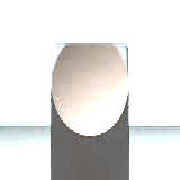
# Autodesk Inventor part: ISO 3601-1 - C 0300 G
Saved by Autodesk Inventor 2021.3 (Build 253353000, 353)
## iProperties
Created: 2020-01-21
Part Number: ISO 3601-1 - C 0300 G
Material: Rubber
Description: Fluid power systems - O-ring
Document SubType Name: Modeling
Standard: ISO 3601-1
Designer: Rémi Heredero
Standard Revision: Third edition 2002-08-01
Standards Organization: ISO
Language: en-US
Size Designation: C 0300 G
Categories: <MemberInstance><Categories><Category DisplayName="Shaft Parts" InternalName="7f7aeb1f-a693-4053-b835-cee3144e0d98" Mnemonic="SHFT"><Category DisplayName="Sealing" InternalName="7cc80d44-b28a-4eb5-95d8-e54d452fb95e" Mnemonic="GSKT"><Category DisplayName="O-Rings" InternalName="33c545bb-13c8-4826-80bf-0503e1d122a8" Mnemonic="ORGSKT"><CategoryParameter DisplayName="O-Ring Inside Diameter" InternalName="2396c6fe-eaf5-4a08-901f-879cfa8d6861" Mnemonic="oindia"/><CategoryParameter DisplayName="O-Ring Cross Section Diameter" InternalName="55cd1771-6829-4a36-adef-b3bef9abff47" Mnemonic="osecdia"/><CategoryParameter DisplayName="Shaft Diameter" InternalName="800cb856-dfd5-475b-a5f5-7930e1c24170" Mnemonic="shaftdia"/><CategoryParameter DisplayName="Thickness" InternalName="d722c673-2dd1-4ecb-b1b2-67404f2aea42" Mnemonic="thick"/><Category DisplayName="Radial Internal" InternalName="94bce4a4-c701-4512-9012-7d41da09bb5a" Mnemonic="ORGSKTRI"><CategoryParameter DisplayName="Groove Width" InternalName="20e3f4bb-a411-4064-be96-21e607b7e471" Mnemonic="NB"/><CategoryParameter DisplayName="Outside Radius" InternalName="58031890-5a64-4422-90a4-8f170607bbac" Mnemonic="R2"/><CategoryParameter DisplayName="Groove Diameter" InternalName="9b90a319-4acb-4bb6-b120-7b7d5fa3e797" Mnemonic="NDOR"/><CategoryParameter DisplayName="Inside Radius" InternalName="cafdab84-b5be-4c6a-8c01-58bfed4b804b" Mnemonic="R1"/></Category></Category></Category></Category><Category DisplayName="DataType" InternalName="23b78d0f-2648-40c6-8793-ca6db495c9e8" Mnemonic="DATATYPE"><CategoryParameter DisplayName="DisplayName" InternalName="05415f3d-3907-474b-a020-eb9d644f4cf3" Mnemonic="DISPLAYNAME"/><CategoryParameter DisplayName="Standard" InternalName="0c0a119c-1e12-4c84-803f-101930972f5e" Mnemonic="STANDARD"/><CategoryParameter DisplayName="Description" InternalName="13903e3d-64b1-4950-80da-f627842ea37f" Mnemonic="DESCRIPTION"/><CategoryParameter DisplayName="Designation" InternalName="2675968c-4ce5-49e0-a4f5-552d29089031" Mnemonic="DESIGNATION"/><CategoryParameter DisplayName="Default Row" InternalName="2af9ec52-faaa-4026-b378-f9fa4afca842" Mnemonic="DEFAULTROW"/><CategoryParameter DisplayName="Folder Name" InternalName="3f06958e-8713-4116-9be7-ed6184ecc97b" Mnemonic="FOLDERNAME"/><CategoryParameter DisplayName="Revision Guid" InternalName="45a75005-10b1-4dfc-8d6d-dfe629f0b93c" Mnemonic="REVISIONGUID"/><CategoryParameter DisplayName="FileName" InternalName="8b46a4cc-9585-4fed-90c3-899f57e09a73" Mnemonic="FILENAME"/><CategoryParameter DisplayName="StdsOrg" InternalName="8f5914e1-4693-403f-8ab5-d37768198c9d" Mnemonic="STDSORG"/><CategoryParameter DisplayName="Family Version" InternalName="914462f6-6e19-4b14-ba84-155b9680b1d0" Mnemonic="FAMILYREVISION"/><CategoryParameter DisplayName="Standard Revision" InternalName="91d5a463-65c2-4fde-b823-3b7fea5e8e17" Mnemonic="STANDARDREVISION"/><CategoryParameter DisplayName="Member Revision" InternalName="a65d44b9-392f-4f4f-857b-e4b3d54996fe" Mnemonic="MEMBERREVISION"/><CategoryParameter DisplayName="ClipFormat" InternalName="bc51e27b-3422-4e78-93ef-cec197ddf230" Mnemonic="CLIPFORMAT"/><CategoryParameter DisplayName="Manufacturer" InternalName="cd6c7a72-a28a-4e50-99a9-2c7f4e13e5ad" Mnemonic="MANUFACTURER"/><CategoryParameter DisplayName="InternalName" InternalName="cf1d0246-76d9-4b4a-8305-fa0409afb5c1" Mnemonic="INTERNALNAME"/><CategoryParameter DisplayName="IsMetric" InternalName="e2385c5b-1ea4-4823-96a8-8de651266ec3" Mnemonic="ISMETRIC"/><Category DisplayName="Part" InternalName="c0e0b642-3bcb-4cc8-9e80-f96d35c4afa4" Mnemonic="PART"><CategoryParameter DisplayName="Part Number" InternalName="016b6077-bfbe-49bd-92c9-d8d59c39c941" Mnemonic="PARTNUMBER"/><CategoryParameter DisplayName="Stock Number" InternalName="4dba7c1c-e26c-444e-836c-b08b433409a8" Mnemonic="STOCKNUMBER"/><CategoryParameter DisplayName="Material Key" InternalName="5c9a8adb-dd2b-4535-b97f-0a94a95fe41f" Mnemonic="MATERIALKEY"/><CategoryParameter DisplayName="Material" InternalName="818a152a-d3c3-49ca-80ee-df7d91421b8e" Mnemonic="MATERIAL"/></Category></Category><Category DisplayName="LegacyMap" InternalName="cd87c42b-3e48-431e-b5c0-1cbeb14dfe77" Mnemonic="LEGACYMAP"><CategoryParameter DisplayName="unique DA member ID" InternalName="0918ad47-427f-4fed-ae26-24c81c58f590" Mnemonic="DACOOKIE"/><CategoryParameter DisplayName="Merge11 ID" InternalName="0ee8fb18-e2ed-4f39-96f6-1f4b5f50aa71" Mnemonic="MERGE11"/><CategoryParameter DisplayName="unique CC member ID" InternalName="5193edd4-b2b0-4ab4-9d54-de900eee34e0" Mnemonic="CCCOOKIE"/><CategoryParameter DisplayName="Split ID" InternalName="72b5c83c-be7f-45c4-ae51-9160ea6deb26" Mnemonic="SPLIT"/><CategoryParameter DisplayName="MemberID" InternalName="8e5e0294-fc51-4c8f-b3d7-003dc5ed94f6" Mnemonic="MEMBERID"/><CategoryParameter DisplayName="CatalogName" InternalName="d99d1e27-aa94-4de2-af4c-c348882a6f4f" Mnemonic="CATALOGNAME"/><CategoryParameter DisplayName="FamilyNumber" InternalName="e705e1f4-09cb-413e-91f9-551b4188271e" Mnemonic="FAMILYNUMBER"/></Category></Categories><FamilyTemplate Id="si0119"><FamilyTemplateParameters><FamilyTemplateParameter ObjectType="kUserParameterObject" ValueType="xs:double" Id="1" ObjectReferenceKey="R1"/><FamilyTemplateParameter ObjectType="kUserParameterObject" ValueType="xs:double" Id="2" ObjectReferenceKey="R2"/><FamilyTemplateParameter ObjectType="kUserParameterObject" ValueType="xs:double" Id="3" ObjectReferenceKey="QDM"/><FamilyTemplateParameter ObjectType="kUserParameterObject" ValueType="xs:double" Id="4" ObjectReferenceKey="SD1"/><FamilyTemplateParameter ObjectType="kUserParameterObject" ValueType="xs:double" Id="5" ObjectReferenceKey="NDOR"/><FamilyTemplateParameter ObjectType="kUserParameterObject" ValueType="xs:double" Id="6" ObjectReferenceKey="NB1"/><FamilyTemplateParameter ObjectType="kUserParameterObject" ValueType="xs:double" Id="7" ObjectReferenceKey="BD"/><FamilyTemplateParameter ObjectType="kUserParameterObject" ValueType="xs:double" Id="8" ObjectReferenceKey="NND"/><FamilyTemplateParameter ObjectType="kUserParameterObject" ValueType="xs:double" Id="120" ObjectReferenceKey="NTOR"/><FamilyTemplateParameter ObjectType="kPropertyObject" ValueType="xs:string" Id="100" ObjectReferenceKey="{32853F0F-3444-11d1-9E93-0060B03C1CA6}" SubObjectId="52"/><FamilyTemplateParameter ObjectType="kPropertyObject" ValueType="xs:string" Id="105" ObjectReferenceKey="{32853F0F-3444-11d1-9E93-0060B03C1CA6}" SubObjectId="5"/><FamilyTemplateParameter ObjectType="kPartComponentDefinitionObject" ValueType="xs:string" Id="110" SubObjectId="Material"/></FamilyTemplateParameters></FamilyTemplate><CategoryParameterMap><ParamToTemplateMap><ParamToTemplate CategoryParameter="//CategoryParameter[@InternalName='05415f3d-3907-474b-a020-eb9d644f4cf3']" ConstantValue="ISO 3601-1 pneumatic"/><ParamToTemplate CategoryParameter="//CategoryParameter[@InternalName='cf1d0246-76d9-4b4a-8305-fa0409afb5c1']" ConstantValue="9b183574-971f-4937-a3ee-caec61f98283"/><ParamToTemplate CategoryParameter="//CategoryParameter[@InternalName='3f06958e-8713-4116-9be7-ed6184ecc97b']" ConstantValue="ISO 3601-1(8)"/><ParamToTemplate CategoryParameter="//CategoryParameter[@InternalName='914462f6-6e19-4b14-ba84-155b9680b1d0']" ConstantValue="10"/><ParamToTemplate CategoryParameter="//CategoryParameter[@InternalName='bc51e27b-3422-4e78-93ef-cec197ddf230']" ConstantValue="CF_INVENTOR.STDPARTS"/><ParamToTemplate CategoryParameter="//CategoryParameter[@InternalName='e2385c5b-1ea4-4823-96a8-8de651266ec3']" ConstantValue="true"/><ParamToTemplate CategoryParameter="//CategoryParameter[@InternalName='13903e3d-64b1-4950-80da-f627842ea37f']" ConstantValue="Fluid power systems - O-ring"/><ParamToTemplate CategoryParameter="//CategoryParameter[@InternalName='8f5914e1-4693-403f-8ab5-d37768198c9d']" ConstantValue="ISO"/><ParamToTemplate CategoryParameter="//CategoryParameter[@InternalName='0c0a119c-1e12-4c84-803f-101930972f5e']" ConstantValue="ISO 3601-1"/><ParamToTemplate CategoryParameter="//CategoryParameter[@InternalName='cd6c7a72-a28a-4e50-99a9-2c7f4e13e5ad']" TemplateParameter="104"/><ParamToTemplate CategoryParameter="//CategoryParameter[@InternalName='91d5a463-65c2-4fde-b823-3b7fea5e8e17']" ConstantValue="Third edition 2002-08-01"/><ParamToTemplate CategoryParameter="//CategoryParameter[@InternalName='45a75005-10b1-4dfc-8d6d-dfe629f0b93c']" ConstantValue="ada2eeba-7769-4b09-87a6-a6832d203b67"/><ParamToTemplate CategoryParameter="//CategoryParameter[@InternalName='2af9ec52-faaa-4026-b378-f9fa4afca842']" ConstantValue="10"/><ParamToTemplate CategoryParameter="//CategoryParameter[@InternalName='d99d1e27-aa94-4de2-af4c-c348882a6f4f']" ConstantValue="ISO"/><ParamToTemplate CategoryParameter="//CategoryParameter[@InternalName='e705e1f4-09cb-413e-91f9-551b4188271e']" ConstantValue="126"/><ParamToTemplate CategoryParameter="//CategoryParameter[@InternalName='8b46a4cc-9585-4fed-90c3-899f57e09a73']" ConstantValue="ISO 3601-1 - C 0300 G 30(8)"/><ParamToTemplate CategoryParameter="//CategoryParameter[@InternalName='a65d44b9-392f-4f4f-857b-e4b3d54996fe']" ConstantValue="9DB31403-C1F9-4E75-A126-2D4390AC9453"/><ParamToTemplate CategoryParameter="//CategoryParameter[@InternalName='8e5e0294-fc51-4c8f-b3d7-003dc5ed94f6']" ConstantValue="540"/><ParamToTemplate CategoryParameter="//CategoryParameter[@InternalName='2675968c-4ce5-49e0-a4f5-552d29089031']" TemplateParameter="100"/><ParamToTemplate CategoryParameter="//CategoryParameter[@InternalName='818a152a-d3c3-49ca-80ee-df7d91421b8e']" TemplateParameter="110"/><ParamToTemplate CategoryParameter="//CategoryParameter[@InternalName='20e3f4bb-a411-4064-be96-21e607b7e471']" TemplateParameter="6"/><ParamToTemplate CategoryParameter="//CategoryParameter[@InternalName='9b90a319-4acb-4bb6-b120-7b7d5fa3e797']" TemplateParameter="5"/><ParamToTemplate CategoryParameter="//CategoryParameter[@InternalName='800cb856-dfd5-475b-a5f5-7930e1c24170']" TemplateParameter="8"/><ParamToTemplate CategoryParameter="//CategoryParameter[@InternalName='d722c673-2dd1-4ecb-b1b2-67404f2aea42']" TemplateParameter="120"/><ParamToTemplate CategoryParameter="//CategoryParameter[@InternalName='016b6077-bfbe-49bd-92c9-d8d59c39c941']" TemplateParameter="105"/><ParamToTemplate CategoryParameter="//CategoryParameter[@InternalName='55cd1771-6829-4a36-adef-b3bef9abff47']" TemplateParameter="3"/><ParamToTemplate CategoryParameter="//CategoryParameter[@InternalName='cafdab84-b5be-4c6a-8c01-58bfed4b804b']" TemplateParameter="1"/><ParamToTemplate CategoryParameter="//CategoryParameter[@InternalName='58031890-5a64-4422-90a4-8f170607bbac']" TemplateParameter="2"/><ParamToTemplate CategoryParameter="//CategoryParameter[@InternalName='2396c6fe-eaf5-4a08-901f-879cfa8d6861']" TemplateParameter="4"/></ParamToTemplateMap></CategoryParameterMap></MemberInstance>
Density: 0.93 g/cm^3
Appearance: Rubber - Black
IsCustomPart: 0
Author: Rémi Heredero
Autodesk Inventor part; units mm, degrees
ref_plane "YZ Plane" through (0, 0, 0) normal (1, 0, 0) x (0, 1, 0)
ref_plane "XZ Plane" through (0, 0, 0) normal (0, 1, 0) x (-1, 0, 0)
ref_plane "XY Plane" through (0, 0, 0) normal (0, 0, 1) x (1, 0, 0)
sketch "Sketch1" plane through (0, 0, 0) normal (0, 0, 1) x (1, 0, 0)
  line L0 (-0.0113, 0) -> (-0.0113, 0) construction
  line L1 (-0.7685, 3.2) -> (0.7685, 3.2)
  line L2 (-0.7685, 0) -> (0.7685, 0)
  arc A0 (-0.7685, 3.2) -> (-0.7685, 0) centre (0, 1.6) ccw
  line L3 (-4, -15) -> (6.0335, -15)
  line L4 (-6.0067, 0) -> (8.0403, 0) projected
  line L5 (0, 4.64) -> (0, -12.44) projected
  arc A1 (0.7685, 0) -> (0.7685, 3.2) centre (0, 1.6) ccw
  dimension "d0" = 30
  dimension "d1" = 1.6
  dimension "d2" = 1.775
  dimension "d3" = 1.6
  dimension "d4" = 3.2
  constraints: 8 end point, 4 point on circle, 2 centre point, 2 horizontal alignment, 2 parallel, 1 coincident, 1 horizontal, 1 point on line, 1 other
  measures "d0" diameter of L4 L3
  measures "d1" distance from line of A0.centre L1
  measures "d2" radius of A0
  measures "d3" distance from line of L2 A0.centre
  measures "d4" distance between parallel lines of L4 L1
revolve "Body" add sketch "Sketch1" angle 360 about axis through (-4, -15, 0) along (1, 0, 0)
equation "\"d0\" = NND"
equation "\"d1\" = -0.25 * NND + 0.25 * NDOR"
equation "\"d2\" = 0.5 * QDM"
equation "\"d3\" = -0.25 * NND + 0.25 * NDOR"
equation "\"d4\" = -0.5 * NND + 0.5 * NDOR"
equation "\"QDM\" = 3.55"
equation "\"NND\" = 30"
equation "\"NDOR\" = 36.4"
equation "\"R1\" = 0.6"
equation "\"R2\" = 0.2"
equation "\"NB1\" = 4.6"
equation "\"BD\" = 30.15"
equation "\"NTOR\" = -0.5 * NND + 0.5 * NDOR"
body "Solid1"
